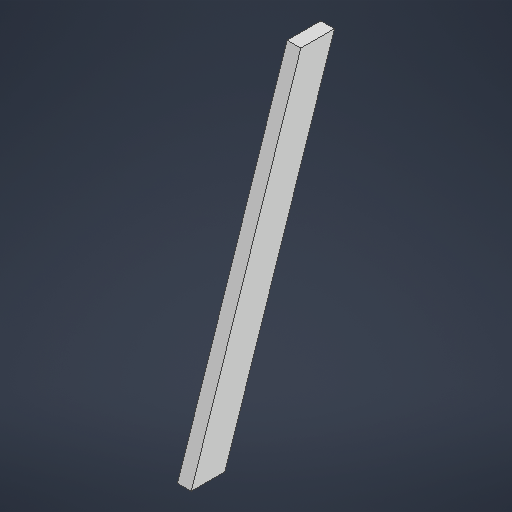
# Autodesk Inventor part: taildiag
Saved by Autodesk Inventor 2027.1 (Build 311270010, 270A)
## iProperties
Created: 2026-09-04
Part Number: taildiag
Material: Generic
Document SubType Name: Modeling
Designer: jorda
Density: 1 g/cm^3
Appearance: Default
Author: jorda
Autodesk Inventor part; units mm, degrees
ref_plane "YZ Plane" through (0, 0, 0) normal (1, 0, 0) x (0, 1, 0)
ref_plane "XZ Plane" through (0, 0, 0) normal (0, 1, 0) x (-1, 0, 0)
ref_plane "XY Plane" through (0, 0, 0) normal (0, 0, 1) x (1, 0, 0)
sketch "Sketch1" plane through (0, 0, 0) normal (1, 0, 0) x (0, 1, 0)
  line L0 (0, -93.7088) -> (0, 0)
  line L1 (0, 0) -> (914.4, -304.8)
  line L2 (886.2874, -389.1379) -> (633.2735, -304.8)
  line L3 (914.4, -304.8) -> (914.4, -398.5088)
  line L4 (832.31, -371.1455) -> (886.2874, -389.1379)
  line L5 (633.2735, -304.8) -> (0, -93.7088)
  line L6 (886.2874, -389.1379) -> (914.4, -398.5088)
  constraints: 14 end point, 1 point on line, 1 vertical
extrude "Extrusion1" add sketch "Sketch1" along normal blind 38.1
body "Solid1"
